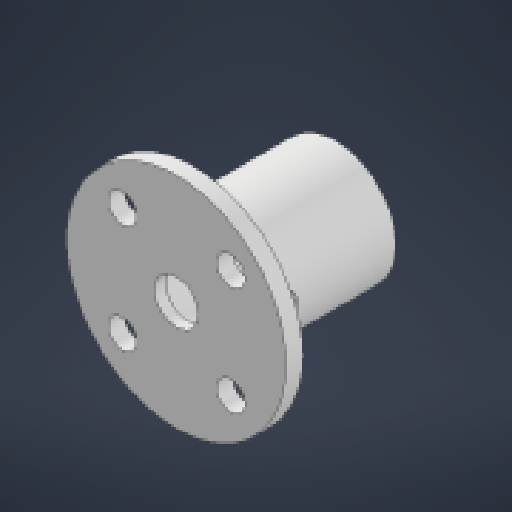
# Autodesk Inventor part: motor_clamp
Saved by Autodesk Inventor 2026.1 (Build 301233020, 233B)
## iProperties
Created: 2025-11-21
Part Number: motor_clamp
Material: 일반
Document SubType Name: Modeling
Designer: jaewook
Density: 1 g/cm^3
Appearance: 기본값
Author: jaewook
Autodesk Inventor part; units mm, degrees
ref_plane "YZ Plane" through (0, 0, 0) normal (1, 0, 0) x (0, 1, 0)
ref_plane "XZ Plane" through (0, 0, 0) normal (0, 1, 0) x (-1, 0, 0)
ref_plane "XY Plane" through (0, 0, 0) normal (0, 0, 1) x (1, 0, 0)
sketch "스케치1" plane through (0, 0, 0) normal (0, 0, 1) x (1, 0, 0)
  circle A0 centre (0.5479, -1.5474) radius 5.5
  circle A1 centre (0.5479, -1.5474) radius 5
  circle A2 centre (0.5479, -1.5474) radius 4.2
  ellipse E0 centre (0.5479, -1.5474) end of major axis (-0.0909, -9.0201) minor radius 7.4992
  ellipse E1 centre (0.5479, -1.5474) end of major axis (-0.0912, -9.0201) minor radius 7.4991
  ellipse E2 centre (0.5479, -1.5474) end of major axis (1.2999, 2.3813) minor radius 3.9993 (-3.4513, -1.5143) -> (4.5471, -1.5804) ccw projected
  dimension "d0" = 10
  dimension "d1" = 8.4
  dimension "d24" = 11
  constraints: 5 coincident, 3 centre point, 5 other
  measures "d0" diameter of A1
  measures "d1" diameter of A2
  measures "d24" diameter of A0
extrude "돌출1" add sketch "스케치1" against normal blind 8 contours A1
sketch "스케치2" plane through (0.5479, -1.5474, 0) normal (0, 0, 1) x (1, 0, 0)
  circle A0 centre (0, 0) radius 4.2 projected
  circle A1 centre (0, 0) radius 5.5
  dimension "d4" = 11
  constraints: 1 centre point, 1 coincident
  measures "d4" diameter of A1
extrude "돌출2" add sketch "스케치2" along normal blind 5
sketch "스케치3" plane through (0.5479, -1.5474, 5) normal (0, 0, 1) x (1, 0, 0)
  circle A0 centre (0, 0) radius 5.5 projected
  circle A1 centre (0, 0) radius 4.2 projected
  circle A2 centre (0, 0) radius 10
  circle A3 centre (4.9497, -4.9497) radius 1.3
  circle A4 centre (0, 0) radius 5 projected
  line L0 (0, 0) -> (0, -5.5) construction
  circle A5 centre (4.9497, 4.9497) radius 1.3
  circle A6 centre (-4.9497, 4.9497) radius 1.3
  circle A7 centre (-4.9497, -4.9497) radius 1.3
  dimension "d9" = 20
  dimension "d10" = 2.6
  dimension "d11" = 7
  dimension "d12" = 45
  dimension "d15" = 360
  constraints: 5 centre point, 2 end point, 1 coincident, 1 vertical, 1 vertical alignment, 10 other
  measures "d9" diameter of A2
  measures "d10" diameter of A3
  measures "d11" distance of point (0, 0) A3.centre
extrude "돌출3" add sketch "스케치3" along normal blind 1.5 contours A0 | A2 | A4
sketch "스케치4" plane through (0.5479, -1.5474, 6.5) normal (0, 0, 1) x (1, 0, 0)
  circle A0 centre (0, 0) radius 4.2 projected
  circle A1 centre (0, 0) radius 2
  dimension "d17" = 4
  constraints: 1 centre point, 1 coincident
  measures "d17" diameter of A1
extrude "돌출4" add sketch "스케치4" against normal blind 1
sketch "스케치5" plane through (0, 0, 0) normal (1, 0, 0) x (0, 1, 0)
  circle A0 centre (-1.5474, 2.5) radius 1.5
  line L0 (3.9526, 0) -> (-7.0474, 0) projected
  line L1 (3.9526, 5) -> (-7.0474, 5) projected
  line L2 (3.9526, 0) -> (-7.0474, 0) projected
  line L3 (-7.0474, 0) -> (-7.0474, 5) projected
  line L4 (3.9526, 0) -> (3.9526, 5) projected
  point P0 (0, 0)
  point P1 (-1.5474, 5)
  dimension "d20" = 3
  dimension "d21" = 2.5
  constraints: 1 centre point, 1 midpoint, 1 vertical alignment
  measures "d20" diameter of A0
  measures "d21" distance from line of L0 A0.centre
extrude "돌출5" cut sketch "스케치5" along normal through all both and the other way through all contours A0
sketch "스케치6" plane through (0.5479, -1.5474, 0) normal (0, 0, -1) x (-1, 0, 0)
  circle A0 centre (0, 0) radius 5.5 projected
  circle A1 centre (0, 0) radius 5 projected
  point P0 (0.5479, 1.5474)
extrude "돌출6" add sketch "스케치6" along normal blind 8
